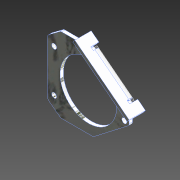
# Autodesk Inventor part: trackball-cover
Saved by Autodesk Inventor 2018 (Build 220112000, 112)
## iProperties
Created: 2018-06-15
Part Number: trackball-cover
Material: アルミニウム 6061
Document SubType Name: Sheet Metal
Designer: NaMACHAN
Density: 2.7 g/cm^3
Sheet Metal Rule: Default
Appearance: アルミニウム - フラット
Mass: 3.65827 g
Surface Area: 22.6789 cm^2
Volume: 1.35491 cm^3
Author: NaMACHAN
Autodesk Inventor part; units mm, degrees
ref_plane "YZ Plane" through (0, 0, 0) normal (1, 0, 0) x (0, 1, 0)
ref_plane "XZ Plane" through (0, 0, 0) normal (0, 1, 0) x (-1, 0, 0)
ref_plane "XY Plane" through (0, 0, 0) normal (0, 0, 1) x (1, 0, 0)
sketch "スケッチ8" plane through (0, 0, 0) normal (0, 1, 0) x (-1, 0, 0)
  line L0 (0, 0) -> (-8, -6)
  line L1 (-8, -6) -> (-28, -6)
  line L2 (-28, -6) -> (-50, 11)
  line L3 (-50, 11) -> (-50, 23)
  line L4 (-50, 23) -> (-28, 40)
  line L5 (-28, 40) -> (-8, 40)
  line L6 (-8, 40) -> (0, 34)
  line L7 (0, 34) -> (0, 0)
  circle A0 centre (-25, 17) radius 17.35
  dimension "d41" = 34
  dimension "d42" = 6
  dimension "d43" = 6
  dimension "d44" = 8
  dimension "d45" = 20
  dimension "d46" = 22
  dimension "d47" = 17
  dimension "d48" = 17
  dimension "d49" = 34.7
  dimension "d50" = 25
  dimension "d51" = 23
  measures "d41" distance of L0.start L6.end
  measures "d42" vertical distance of L0.end L0.start
  measures "d43" vertical distance of L5.end L6.end
  measures "d44" horizontal distance of L5.end L6.end
  measures "d45" distance of L4.end L5.end
  measures "d46" horizontal distance of L3.end L4.end
  measures "d47" distance from line of L1 L2.end
  measures "d48" distance from line of L3.end L5
  measures "d49" diameter of A0
  measures "d50" distance from line of L7 A0.centre
  measures "d51" distance from line of L1 A0.centre
extrude "プレート6" add sketch "スケッチ8" along normal blind 2
sketch "スケッチ9" plane through (0, 2, 0) normal (0, 1, 0) x (1, 0, 0)
  line L0 (0, -34) -> (0, 0) projected
  line L1 (50, -11) -> (50, -23) projected
  point P0 (4, -4)
  point P1 (4, -30)
  point P2 (47, -22)
  point P3 (47, -12)
  dimension "d53" = 4
  dimension "d54" = 4
  dimension "d55" = 26
  dimension "d56" = 3
  dimension "d57" = 1
  dimension "d58" = 1
  constraints: 2 vertical alignment
  measures "d53" distance from line of L0 point (4, -4)
  measures "d54" horizontal distance of L0.start point (4, -30)
  measures "d55" distance of point (4, -4) point (4, -30)
  measures "d56" distance from line of L1 point (47, -12)
  measures "d57" vertical distance of L1.start point (47, -12)
  measures "d58" vertical distance of L1.end point (47, -22)
hole "穴1" at (4, 2, 4) at (4, 2, 30) at (47, 2, 22) at (47, 2, 12) direction (0, -1, 0) diameter 3 end through all
fillet "コーナーR1" radius 2 8 edges at (0, 1, 34) (8, 1, 40) (28, 1, 40) (50, 1, 23) (50, 1, 11) (28, 1, -6) (0, 1, 0) (8, 1, -6)
sketch "スケッチ10" plane through (49.2229, 0, 23.6005) normal (0.6114475, 0, 0.791285) x (0.791285, 0, -0.6114475)
  point P0 (-24.5189, 0)
equation "\"d64\" = Thickness"
equation "\"d52\" = Thickness"
equation "\"BendRadius\" = Thickness"
equation "\"BendReliefWidth\" = Thickness"
equation "\"BendReliefDepth\" = 0.5 * Thickness"
equation "\"CornerReliefSize\" = 4 * Thickness"
equation "\"MinimumRemnant\" = 2 * Thickness"
equation "\"TransitionRadius\" = BendRadius"
equation "\"JacobiRadiusSize\" = Thickness"
equation "\"GapSize\" = Thickness"
equation "\"Thickness\" = 2"
